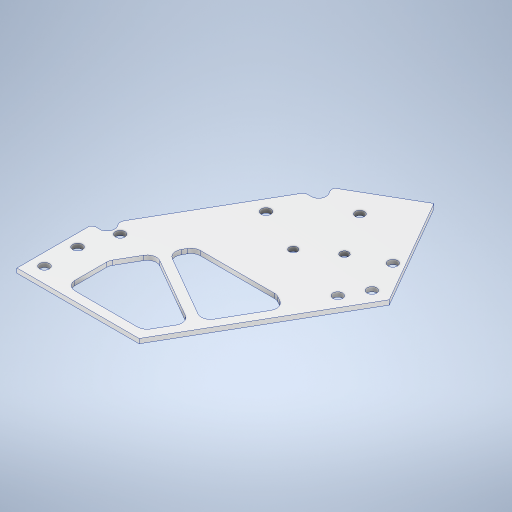
# Autodesk Inventor part: base_base
Saved by Autodesk Inventor 2024.1 (Build 281209000, 209)
## iProperties
Created: 2025-01-17
Part Number: base_base
Material: アルミニウム 6061
Document SubType Name: Sheet Metal
Designer: hibik
Density: 2.7 g/cm^3
Sheet Metal Rule: Default_mm
Appearance: アルミニウム - フラット
Author: hibik
Autodesk Inventor part; units mm, degrees
ref_plane "YZ Plane" through (0, 0, 0) normal (1, 0, 0) x (0, 1, 0)
ref_plane "XZ Plane" through (0, 0, 0) normal (0, 1, 0) x (-1, 0, 0)
ref_plane "XY Plane" through (0, 0, 0) normal (0, 0, 1) x (1, 0, 0)
sketch "スケッチ2" plane through (0, 0, 0) normal (0, 1, 0) x (-1, 0, 0)
  line L0 (0, 0) -> (40, 0)
  line L1 (40, 0) -> (40, -23.7735)
  line L2 (-30, -51.9615) -> (0, 0)
  line L3 (-30, -51.9615) -> (-10, -86.6025)
  line L4 (-10, -86.6025) -> (10.5885, -74.7158)
  line L5 (10.5885, -74.7158) -> (40, -23.7735)
  line L6 (-30, -51.9615) -> (-36.3397, -48.3013) construction
  line L7 (30, 0) -> (30, -18) construction
  line L8 (30, -18) -> (40, -23.7735) construction
  dimension "d0" = 60
  dimension "d1" = 60
  dimension "d2" = 40
  dimension "d3" = 60
  dimension "d4" = 18
  dimension "d5" = 30
  dimension "d6" = 60
  measures "d0" angle of L0 L2
  measures "d1" angle of L2 L3
  measures "d2" distance of L0.start L0.end
  measures "d3" distance from line of L0.start L6
  measures "d4" distance of L7.start L7.end
  measures "d5" distance from line of L0.start L7
  measures "d6" angle of L7 L8
extrude "プレート1" add sketch "スケッチ2" along normal blind 1.5
sketch "スケッチ3" plane through (0, 1.5, 0) normal (0, 1, 0) x (1, 0, 0)
  line L0 (-10.5885, 74.7158) -> (-40, 23.7735) projected
  line L1 (-31.7863, 38) -> (10.9697, 38)
  line L2 (10.9697, 38) -> (19.1969, 33.25)
  line L3 (0, 0) -> (30, 51.9615) projected
  line L4 (30, 51.9615) -> (0, 0) projected
  line L5 (0, 0) -> (-40, 0) projected
  circle A0 centre (0, 50.5) radius 12.5 construction
  circle A1 centre (0, 50.5) radius 1.35
  circle A2 centre (0, 50.5) radius 10.5 construction
  circle A3 centre (0.8246, 71.4838) radius 10.5 construction
  circle A4 centre (0.8246, 71.4838) radius 11.5 construction
  line L6 (10, 86.6025) -> (30, 51.9615) projected
  circle A5 centre (0.8246, 71.4838) radius 1.5
  line L7 (-30, 0) -> (-30, 18)
  line L8 (-30, 18) -> (-18.453, 38)
  line L9 (-40, 23.7735) -> (-10.5885, 74.7158) projected
  line L10 (-31.3397, 18.7735) -> (-1.9282, 69.7158)
  line L11 (-1.9282, 69.7158) -> (-10.5885, 74.7158)
  line L12 (-40, 23.7735) -> (-40, 0) projected
  line L13 (-40, 23.7735) -> (-30, 18)
  line L14 (-21.1225, 56.4702) -> (-12.4623, 51.4702)
  circle A6 centre (9.6953, 57.5712) radius 6 construction
  circle A7 centre (0, 50.5) radius 6 construction
  circle A8 centre (9.6953, 57.5712) radius 1.35
  dimension "d10" = 25
  dimension "d8" = 38
  dimension "d9" = 9.5
  dimension "d11" = 2.7
  dimension "d14" = 21
  dimension "d15" = 21
  dimension "d16" = 23
  dimension "d17" = 3
  dimension "d18" = 30
  dimension "d19" = 18
  dimension "d20" = 10
  dimension "d37" = 2.7
  dimension "d38" = 12
  constraints: 16 end point, 8 centre point, 7 point on line, 6 coincident, 3 equal radius, 3 parallel, 2 horizontal, 2 perpendicular, 2 tangent, 1 vertical, 1 vertical alignment, 3 other
  measures "d8" distance between parallel lines of L5 L1
  measures "d9" distance from line of L1.end L3
  measures "d11" diameter of A1
  measures "d14" diameter of A2
  measures "d15" diameter of A3
  measures "d16" diameter of A4
  measures "d17" diameter of A5
  measures "d18" distance from line of L3.start L7
  measures "d19" distance of L7.start L7.end
  measures "d20" distance between parallel lines of L0 L10
  measures "d37" diameter of A8
  measures "d38" diameter of A7
extrude "切り取り1" cut sketch "スケッチ3" against normal blind 1.5 contours A1 | A5 | A8
sketch "スケッチ4" plane through (0, 1.5, 0) normal (0, 1, 0) x (1, 0, 0)
  circle A0 centre (-36, 5) radius 1.6 projected
  circle A1 centre (-36, 15.8638) radius 1.6 projected
  line L0 (17.129, 44.6683) -> (18.7744, 47.5183) projected
  circle A2 centre (20.4199, 44.6683) radius 1.6 projected
  circle A3 centre (24.5152, 51.7615) radius 1.6 projected
  circle A4 centre (-32.6699, 26.4697) radius 1.6 projected
  circle A5 centre (-15.1699, 56.7805) radius 1.6 projected
  arc A6 (16.826, 59.8957) -> (15.9513, 61.7078) centre (17.5091, 61.3425) ccw projected
  circle A7 centre (20.2171, 62.906) radius 1.6
  line L1 (10, 86.6025) -> (30, 51.9615) projected
  line L2 (17.5091, 61.3425) -> (22.8152, 64.406)
  point P0 (0, 0)
  dimension "d39" = 3.2
  dimension "d40" = 3
  constraints: 2 end point, 2 point on line, 1 centre point, 1 perpendicular
  measures "d39" diameter of A7
  measures "d40" distance from line of L1 A7.centre
extrude "切り取り2" cut sketch "スケッチ4" against normal blind 1.5
sketch "スケッチ5" plane through (0, 0, 0) normal (0, -1, 0) x (1, 0, 0)
  circle A0 centre (-12.1327, -70.9375) radius 2.5
  circle A1 centre (-37.5, -27) radius 2.5
  point P0 (0, 0)
  dimension "d23" = 5
  constraints: 2 centre point, 2 coincident, 1 equal radius, 2 other
  measures "d23" diameter of A0
extrude "切り取り3" cut sketch "スケッチ5" against normal blind 1.5
fillet "フィレット1" radius 2 4 edges at (-39.1971, 0.75, -25.1642) (-36.7587, 0.75, -29.3876) (-13.8297, 0.75, -69.1017) (-11.3914, 0.75, -73.325)
sketch "スケッチ6" plane through (0, 1.5, 0) normal (0, 1, 0) x (1, 0, 0)
  circle A0 centre (0, 50.5) radius 1.35 projected
  line L0 (20.4199, 44.6683) -> (-3.6373, 3)
  line L1 (-3.6373, 3) -> (-32, 3)
  line L2 (-32, 3) -> (-32, 19.6299)
  line L3 (-32, 19.6299) -> (-28.6699, 25.3979)
  line L4 (-28.6699, 25.3979) -> (-28.6699, 37.3979)
  line L5 (-28.6699, 37.3979) -> (-18.9019, 54.3164)
  line L6 (-18.9019, 54.3164) -> (-17.1699, 53.3164)
  line L7 (30, 51.9615) -> (0, 0) projected
  line L8 (0, 0) -> (-40, 0) projected
  line L9 (-40, 0) -> (-40, 23.7735) projected
  line L10 (-35.8476, 30.9657) -> (-14.7409, 67.5236) projected
  circle A1 centre (-32.6699, 26.4697) radius 1.6 projected
  circle A2 centre (-32.6699, 26.4697) radius 4
  circle A3 centre (-15.1699, 56.7805) radius 1.6 projected
  circle A4 centre (-15.1699, 56.7805) radius 4
  circle A5 centre (20.4199, 44.6683) radius 4
  circle A6 centre (20.4199, 44.6683) radius 1.6 projected
  line L11 (10, 86.6025) -> (30, 51.9615) projected
  circle A7 centre (0, 50.5) radius 4
  line L12 (19.3214, 40.822) -> (-1.0984, 46.6538)
  line L13 (-1.5301, 46.8042) -> (-16.7, 53.0848)
  circle A8 centre (-36, 5) radius 1.6 projected
  circle A9 centre (-36, 5) radius 4
  line L14 (-3.6373, 3) -> (-15.3983, 52.5458)
  line L15 (-6.7207, 3) -> (-18.9019, 54.3164)
  line L16 (-32, 6.4641) -> (-10.4908, 18.8825)
  line L17 (-9.7676, 15.8359) -> (-32, 3)
  line L18 (-10.6053, 32.3544) -> (9.1115, 43.7379)
  line L19 (-9.8821, 29.3078) -> (13.1258, 42.5915)
  line L20 (-16.8833, 45.8127) -> (-28.6699, 25.3979)
  line L21 (-15.8741, 41.5609) -> (-32, 13.6299)
  point P0 (18.3581, 41.0972)
  dimension "d27" = 8
  dimension "d28" = 3
  dimension "d29" = 3
  dimension "d30" = 3
  dimension "d31" = 3
  dimension "d32" = 3
  dimension "d33" = 3
  dimension "d34" = 30
  constraints: 34 end point, 11 parallel, 11 point on line, 7 tangent, 4 centre point, 4 coincident, 4 point on circle, 3 equal radius, 1 collinear, 1 concentric, 1 midpoint, 1 perpendicular, 6 other
  measures "d27" diameter of A2
  measures "d28" distance between parallel lines of L8 L1
  measures "d29" distance between parallel lines of L10 L5
  measures "d30" distance between parallel lines of L15 L14
  measures "d31" distance between parallel lines of L21 L20
  measures "d32" distance between parallel lines of L16 L17
  measures "d33" distance between parallel lines of L18 L19
  measures "d34" angle of L1 L17
sketch "スケッチ8" plane through (0, 1.5, 0) normal (0, 1, 0) x (1, 0, 0)
  line L0 (0, 0) -> (-40, 0) projected
  line L1 (-30, 0) -> (-30, 18)
  line L2 (-30, 18) -> (-18.453, 38)
  line L3 (-18.453, 38) -> (10.9697, 38)
  line L4 (10.9697, 38) -> (19.1969, 33.25)
  line L5 (30, 51.9615) -> (0, 0) projected
  line L6 (-27, 3) -> (-27, 17.1962)
  line L7 (-27, 17.1962) -> (-16.7209, 35)
  line L8 (-16.7209, 35) -> (10.1658, 35)
  line L9 (10.1658, 35) -> (15.0988, 32.1519)
  line L10 (15.0988, 32.1519) -> (-1.7321, 3)
  line L11 (-1.7321, 3) -> (-27, 3)
  line L12 (-19.8301, 29.6147) -> (-21.3301, 27.0167)
  line L13 (-21.3301, 27.0167) -> (3.7679, 12.5263)
  line L14 (3.7679, 12.5263) -> (5.2679, 15.1244)
  line L15 (5.2679, 15.1244) -> (-19.8301, 29.6147)
  dimension "d41" = 30
  dimension "d42" = 18
  dimension "d43" = 20
  dimension "d44" = 9.5
  dimension "d45" = 3
  dimension "d46" = 3
  dimension "d47" = 3
  dimension "d48" = 3
  dimension "d49" = 3
  dimension "d50" = 3
  dimension "d51" = 3
  dimension "d52" = 11
  constraints: 28 end point, 7 parallel, 3 perpendicular, 2 collinear, 2 point on line, 2 vertical, 1 horizontal
  measures "d41" distance of L0.start L1.start
  measures "d42" distance of L1.start L1.end
  measures "d43" distance from line of L3 L1.end
  measures "d44" distance from line of L3.end L5
  measures "d45" distance between parallel lines of L5 L10
  measures "d46" distance between parallel lines of L4 L9
  measures "d47" distance between parallel lines of L3 L8
  measures "d48" distance between parallel lines of L2 L7
  measures "d49" distance between parallel lines of L1 L6
  measures "d50" distance between parallel lines of L0 L11
  measures "d51" distance between parallel lines of L15 L13
  measures "d52" distance from line of L10.end L13
extrude "切り取り4" cut sketch "スケッチ8" against normal blind 1.5 contours L6 L7 L13 L10 L11 | L7 L8 L9 L10 L15
fillet "フィレット2" radius 3 10 edges at (-1.7321, 0.75, -3) (-27, 0.75, -3) (-27, 0.75, -17.1962) (-21.3301, 0.75, -27.0167) (3.7679, 0.75, -12.5263) (5.2679, 0.75, -15.1244) (15.0988, 0.75, -32.1519) (10.1658, 0.75, -35) (-16.7209, 0.75, -35) (-19.8301, 0.75, -29.6147)
equation "\"d1\" = d0"
equation "\"d12\" = Thickness"
equation "\"d21\" = Thickness"
equation "\"d24\" = Thickness"
equation "\"d29\" = d28"
equation "\"d30\" = d28"
equation "\"d31\" = d28"
equation "\"d32\" = d28"
equation "\"d33\" = d30"
equation "\"d46\" = d45"
equation "\"d47\" = d45"
equation "\"d48\" = d45"
equation "\"d49\" = d45"
equation "\"d50\" = d45"
equation "\"d51\" = d45"
equation "\"d53\" = Thickness"
equation "\"d7\" = Thickness"
equation "\"BendRadius\" = Thickness"
equation "\"BendReliefWidth\" = Thickness"
equation "\"BendReliefDepth\" = 0.5 * Thickness"
equation "\"CornerReliefSize\" = 4 * Thickness"
equation "\"MinimumRemnant\" = 2 * Thickness"
equation "\"TransitionRadius\" = BendRadius"
equation "\"JacobiRadiusSize\" = BendRadius"
equation "\"GapSize\" = Thickness"
equation "\"Thickness\" = 1.5"
